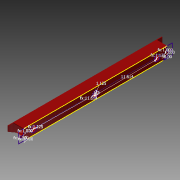
# Autodesk Inventor part: Tube - Right
Saved by Autodesk Inventor 2013 (Build 170138000, 138)
## iProperties
Created: 2013-06-28
Part Number: Tube - Right
Material: Generic
Document SubType Name: Modeling
Designer: mvarma
Density: 1 g/cm^3
Author: mvarma
Autodesk Inventor part; units mm, degrees
ref_plane "YZ Plane" through (0, 0, 0) normal (1, 0, 0) x (0, 1, 0)
ref_plane "XZ Plane" through (0, 0, 0) normal (0, 1, 0) x (-1, 0, 0)
ref_plane "XY Plane" through (0, 0, 0) normal (0, 0, 1) x (1, 0, 0)
sketch "Sketch1" plane through (0, 0, 0) normal (0, 0, 1) x (1, 0, 0)
  line L0 (0, 0) -> (50.8, 0)
  line L1 (50.8, 0) -> (50.8, 50.8)
  line L2 (50.8, 50.8) -> (0, 50.8)
  line L3 (0, 50.8) -> (0, 0)
  line L4 (3.175, 3.175) -> (47.625, 3.175)
  line L5 (47.625, 3.175) -> (47.625, 47.625)
  line L6 (47.625, 47.625) -> (3.175, 47.625)
  line L7 (3.175, 47.625) -> (3.175, 3.175)
  dimension "d0" = 50.8
  dimension "d1" = 50.8
  dimension "d2" = 44.45
  dimension "d3" = 44.45
  dimension "d4" = 3.175
  dimension "d5" = 3.175
  constraints: 16 end point, 4 parallel, 2 horizontal, 2 perpendicular, 1 coincident
  measures "d0" distance of L2.end L1.end
  measures "d1" distance of L1.end L0.end
  measures "d2" distance of L6.end L5.end
  measures "d3" distance of L5.end L4.end
  measures "d4" distance from line of L0 L4.start
  measures "d5" distance between parallel lines of L3 L7
extrude "Extrusion1" add sketch "Sketch1" along normal blind 736.6
sketch "Sketch2" plane through (50.8, 0, 0) normal (1, 0, 0) x (0, 0, -1)
  line L0 (-736.6, 50.8) -> (-711.2, 50.8)
  line L1 (-711.2, 50.8) -> (-711.2, 25.4)
  line L2 (-711.2, 25.4) -> (-736.6, 25.4)
  line L3 (-736.6, 25.4) -> (-736.6, 50.8)
  line L4 (0, 50.8) -> (-25.4, 50.8)
  line L5 (-25.4, 50.8) -> (-25.4, 25.4)
  line L6 (-25.4, 25.4) -> (0, 25.4)
  line L7 (0, 25.4) -> (0, 50.8)
  line L8 (0, 0) -> (-736.6, 0) projected
  line L9 (-736.6, 25.4) -> (-692.6059, 0)
  line L10 (0, 25.4) -> (-43.9941, 0)
  line L11 (0, 0) -> (0, 50.8) projected
  line L12 (-736.6, 0) -> (-736.6, 50.8) projected
  line L13 (-43.9941, 0) -> (0, 0)
  line L14 (0, 25.4) -> (0, 0)
  line L15 (-736.6, 25.4) -> (-736.6, 0)
  line L16 (-692.6059, 0) -> (-736.6, 0)
  line L17 (0, 50.8) -> (-736.6, 50.8) projected
  line L18 (-736.6, 25.4) -> (0, 25.4) construction
  line L19 (-368.3, 50.8) -> (-368.3, 0) construction
  circle A0 centre (-368.3, 22.225) radius 14.2875
  circle A1 centre (-73.3171, 25.4) radius 14.2875
  circle A2 centre (-663.2829, 25.4) radius 14.2875
  dimension "d8" = 25.4
  dimension "d9" = 25.4
  dimension "d10" = 25.4
  dimension "d11" = 25.4
  dimension "d14" = 30
  dimension "d15" = 30
  dimension "d18" = 28.575
  dimension "d19" = 3.175
  dimension "d22" = 295
  dimension "d23" = 28.575
  dimension "d24" = 28.575
  dimension "d25" = 295
  constraints: 32 end point, 5 parallel, 5 point on line, 3 centre point, 3 perpendicular, 2 collinear, 2 horizontal, 2 midpoint
  measures "d8" distance of L1.end L2.end
  measures "d9" distance of L0.end L1.end
  measures "d10" distance of L6.end L5.end
  measures "d11" distance of L5.end L4.end
  measures "d14" angle of L8 L10
  measures "d15" angle of L9 L8
  measures "d18" diameter of A0
  measures "d19" distance from line of L18 A0.centre
  measures "d22" distance of A0.centre A2.centre
  measures "d23" diameter of A2
  measures "d24" diameter of A1
  measures "d25" distance of A1.centre A0.centre
extrude "Extrusion2" cut sketch "Sketch2" against normal up to surface (47.625 mm away) contours L0 L1 L2 L3 | L4 L7 L6 L5
extrude "Extrusion3" cut sketch "Sketch2" against normal through all contours L9 L8 L12 | L10 L11 L8
extrude "Extrusion4" cut sketch "Sketch2" against normal through all contours A0 | A1 | A2
equation "\"d8\" = d9"
equation "\"d9\" = d11"
equation "\"d11\" = d10"
equation "\"d15\" = d14"
equation "\"d22\" = d25"
equation "\"d23\" = d18"
equation "\"d24\" = d18"
body "Solid1"
